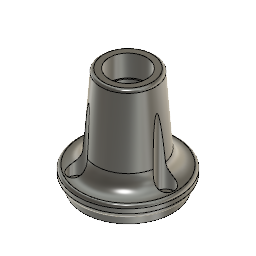
Unterteil-2 (Autodesk Fusion 360 design; units mm, degrees)
Autodesk Fusion 360 part; units mm, degrees
sketch "Skizze1" plane through (0, 0, 0) normal (0, 0, 1) x (1, 0, 0)
  circle A0 centre (0, 0) radius 15.5
  dimension "d1" = 31
  measures "d1" diameter of A0
extrude "Extrusion1" add sketch "Skizze1" along normal blind 2.5
sketch "Skizze2" plane through (0, 0, 2.5) normal (0, 0, 1) x (-1, 0, 0)
  circle A0 centre (0, 0) radius 15.5
  circle A1 centre (0, 0) radius 17.5
  dimension "d4" = 35
  measures "d4" diameter of A1
extrude "Extrusion2" add sketch "Skizze2" along normal blind 4.5 contours A0 | A1
sketch "Skizze3" plane through (0, 0, 7) normal (0, 0, 1) x (-1, 0, 0)
  circle A0 centre (0, 0) radius 17.5
  circle A1 centre (0, 0) radius 11.5
  dimension "d7" = 23
  measures "d7" diameter of A1
ref_plane "Arbeitsebene1" through (0, 0, 41) normal (0, 0, 1) x (-1, 0, 0)
sketch "Skizze4" plane through (0, 0, 41) normal (0, 0, 1) x (1, 0, 0)
  circle A0 centre (0, 0) radius 9
  dimension "d9" = 18
  measures "d9" diameter of A0
loft "Erhebung1" add profiles "Skizze3", "Skizze4" section 1 contours A1 section 2
fillet "Abrundung3" radius 5.5 1 edges at (10.7218, -4.1586, 7)
sketch "Skizze5" plane through (0, 0, 41) normal (0, 0, 1) x (-1, 0, 0)
  circle A0 centre (0, 0) radius 9
  circle A1 centre (0, 0) radius 6
  dimension "d13" = 12
  measures "d13" diameter of A1
extrude "Extrusion3" cut sketch "Skizze5" against normal blind 55 contours A1
sketch "Skizze6" plane through (0, 0, 0) normal (0, 0, -1) x (1, 0, 0)
  circle A0 centre (0, 0) radius 6
  circle A1 centre (0, 0) radius 15.5
  circle A2 centre (0, 0) radius 8.1
  dimension "d16" = 16.2
  measures "d16" diameter of A2
extrude "Extrusion4" cut sketch "Skizze6" against normal blind 9 contours A2
sketch "Skizze7" plane through (0, 0, 0) normal (0, 0, -1) x (1, 0, 0)
  circle A0 centre (0, 0) radius 8.1
  circle A1 centre (0, 0) radius 15.5
  line L0 (-15.5, 0) -> (13, 0)
  circle A2 centre (13, 0) radius 1.6
  circle A3 centre (-6.5, 11.2583) radius 1.6
  circle A4 centre (-6.5, -11.2583) radius 1.6
  dimension "d20" = 3.2
  dimension "d22" = 360
  measures "d20" diameter of A2
extrude "Extrusion5" cut sketch "Skizze7" against normal blind 12 contours A2 | A3 | A4
sketch "Skizze8" plane through (0, 0, 41) normal (0, 0, 1) x (-1, 0, 0)
  circle A0 centre (0, 0) radius 6
  circle A1 centre (0, 0) radius 9
  circle A2 centre (-13, 0) radius 3
  circle A3 centre (6.5, -11.2583) radius 3
  circle A4 centre (6.5, 11.2583) radius 3
  dimension "d25" = 6
  dimension "d27" = 360
  measures "d25" diameter of A2
extrude "Extrusion6" cut sketch "Skizze8" against normal blind 37 contours A2 | A3 | A4
move_face "Flächen versetzen1" offset -5 1 faces at (-7.9442, -0.7452, 41)
fillet "Abrundung5" radius 1 1 edges at (8.7337, -3.3875, 36)
fillet "Abrundung6" radius 1 1 edges at (16.3157, 6.3283, 7)
sketch "Skizze9" plane through (0, 0, 36) normal (0, 0, 1) x (-1, 0, 0)
  circle A0 centre (0, 0) radius 6
  circle A1 centre (0, 0) radius 8.4385
  circle A2 centre (0, 0) radius 6
  circle A3 centre (0, 0) radius 8
  circle A4 centre (0, 0) radius 6.5
  dimension "d34" = 13
  measures "d34" diameter of A4
extrude "Extrusion7" cut sketch "Skizze9" against normal blind 7.5 contours A4
fillet "Abrundung7" radius 2 1 edges at (16.3157, 6.3283, 2.5)
chamfer "Fase3" distance 2 angle 45 1 edges at (5.594, -2.1697, 9)
sketch "Skizze10" plane through (0, 0, 0) normal (0, 0, 1) x (1, 0, 0)
